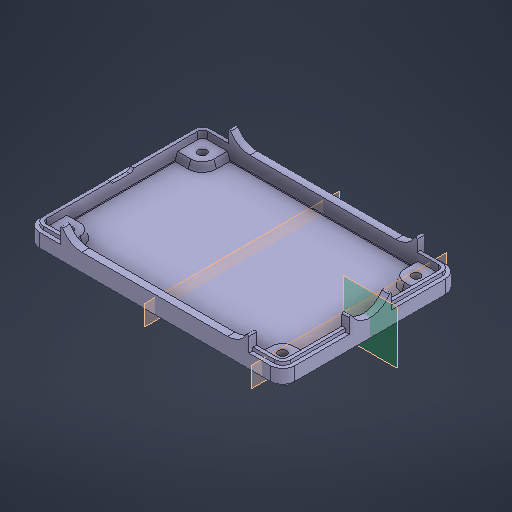
# Autodesk Inventor part: case1
Saved by Autodesk Inventor 2025.2 (Build 292293000, 293)
## iProperties
Created: 2025-10-04
Part Number: case1
Material: Generic
Document SubType Name: Modeling
Designer: micyg
Density: 1 g/cm^3
Appearance: Default
Author: micyg
## iProperties of the stored document case1_3DPrint.ipt
Created: 2025-10-05
Part Number: case1_3DPrint
Material: Generic
Document SubType Name: Modeling
Designer: micyg
Density: 1 g/cm^3
Appearance: Default
Author: micyg
Autodesk Inventor part; units mm, degrees
ref_plane "YZ Plane" through (0, 0, 0) normal (1, 0, 0) x (0, 1, 0)
ref_plane "XZ Plane" through (0, 0, 0) normal (0, 1, 0) x (-1, 0, 0)
ref_plane "XY Plane" through (0, 0, 0) normal (0, 0, 1) x (1, 0, 0)
sketch "Sketch1" plane through (0, 0, 0) normal (0, 1, 0) x (-1, 0, 0)
  line L0 (0, 0) -> (105.2, 0)
  line L1 (105.2, 0) -> (105.2, -72.2)
  line L2 (105.2, -72.2) -> (0, -72.2)
  line L3 (0, -72.2) -> (0, 0)
  line L4 (0, -72.2) -> (105.2, 0) construction
  line L5 (3.6, -3.6) -> (101.6, -3.6) construction
  line L6 (101.6, -3.6) -> (101.6, -68.6) construction
  line L7 (101.6, -68.6) -> (3.6, -68.6) construction
  line L8 (3.6, -68.6) -> (3.6, -3.6) construction
  line L9 (3.6, -3.6) -> (101.6, -68.6) construction
  line L10 (101.6, -3.6) -> (3.6, -68.6) construction
  point P0 (52.6, -36.1)
  dimension "d17" = 98
  dimension "d18" = 65
  dimension "d21" = 72.2
  dimension "d22" = 105.2
  constraints: 22 end point, 4 parallel, 3 midpoint, 2 horizontal, 2 perpendicular
  measures "d17" distance of L6.end L7.end
  measures "d18" distance of L5.end L6.end
  measures "d21" distance between parallel lines of L2 L0
  measures "d22" distance between parallel lines of L3 L1
extrude "Extrusion1" add sketch "Sketch1" along normal blind 7.6
ref_plane "Work Plane7" through (0, 7.6, -36.1) normal (0, 0, -1) x (-1, 0, 0)
fillet "Fillet3" radius 5 4 edges at (-105.2, 3.8, -72.2) (-105.2, 3.8, 0) (0, 3.8, -72.2) (0, 3.8, 0)
chamfer "Chamfer1" distance 2 angle 45 8 edges at (0, 0, -36.1) (-1.4645, 0, -70.7355) (-52.6, 0, -72.2) (-103.7355, 0, -70.7355) (-105.2, 0, -36.1) (-103.7355, 0, -1.4645) (-52.6, 0, 0) (-1.4645, 0, -1.4645)
shell "Shell2" thickness 3 removed faces 1 at (-36.7333, 7.6, -48.1333)
sketch "Sketch2" plane through (-100.2, 3, -69.2) normal (0, 1, 0) x (1, 0, 0)
  line L0 (91.5, -5.6) -> (3.5, -5.6) construction
  line L1 (3.5, -5.6) -> (3.5, -60.6) construction
  line L2 (3.5, -60.6) -> (91.5, -60.6) construction
  line L3 (91.5, -60.6) -> (91.5, -5.6) construction
  arc A0 (91.5, -55.85) -> (86.75, -60.6) centre (91.5, -60.6) ccw
  line L4 (95, 0) -> (0, 0) construction
  arc A1 (-2, -64.2) -> (0, -66.2) centre (0, -64.2) ccw projected
  line L5 (-2, -64.2) -> (-2, -2) projected
  arc A2 (0, 0) -> (-2, -2) centre (0, -2) ccw projected
  line L6 (0, 0) -> (95.2, 0) projected
  arc A3 (97.2, -2) -> (95.2, 0) centre (95.2, -2) ccw projected
  line L7 (97.2, -2) -> (97.2, -64.2) projected
  arc A4 (95.2, -66.2) -> (97.2, -64.2) centre (95.2, -64.2) ccw projected
  line L8 (95.2, -66.2) -> (0, -66.2) projected
  arc A5 (95.2, -69.2) -> (100.2, -64.2) centre (95.2, -64.2) ccw projected
  line L9 (100.2, -64.2) -> (100.2, -2) projected
  arc A6 (100.2, -2) -> (95.2, 3) centre (95.2, -2) ccw projected
  line L10 (95.2, 3) -> (0, 3) projected
  arc A7 (0, 3) -> (-5, -2) centre (0, -2) ccw projected
  line L11 (-5, -2) -> (-5, -64.2) projected
  arc A8 (-5, -64.2) -> (0, -69.2) centre (0, -64.2) ccw projected
  line L12 (0, -69.2) -> (95.2, -69.2) projected
  line L13 (91.5, -55.85) -> (97.2, -55.85)
  line L14 (86.75, -60.6) -> (86.75, -66.2)
  circle A9 centre (91.5, -60.6) radius 1.75
  line L15 (-5, -2) -> (-5, -64.2) projected
  line L16 (-5, -33.1) -> (100.2, -33.1) construction
  line L17 (47.6, -69.2) -> (47.6, 3) construction
  line L18 (3.5, -60.6) -> (91.5, -5.6) construction
  line L19 (47.5, -5.6) -> (47.5, -60.6) construction
  line L20 (-1.5, -0.6) -> (96.5, -0.6) construction
  line L21 (96.5, -0.6) -> (96.5, -65.6) construction
  line L22 (96.5, -65.6) -> (-1.5, -65.6) construction
  line L23 (-1.5, -65.6) -> (-1.5, -0.6) construction
  line L24 (-1.5, -0.6) -> (96.5, -65.6) construction
  arc A10 (86.75, -5.6) -> (91.5, -10.35) centre (91.5, -5.6) ccw
  line L25 (91.5, -10.35) -> (97.2, -10.35)
  line L26 (86.75, -5.6) -> (86.75, 0)
  circle A11 centre (91.5, -5.6) radius 1.75
  arc A12 (8.25, -60.6) -> (3.5, -55.85) centre (3.5, -60.6) ccw
  line L27 (8.25, -60.6) -> (8.25, -66.2)
  circle A13 centre (3.5, -60.6) radius 1.75
  arc A14 (3.5, -10.35) -> (8.25, -5.6) centre (3.5, -5.6) ccw
  line L28 (8.25, -5.6) -> (8.25, 0)
  circle A15 centre (3.5, -5.6) radius 1.75
  line L29 (3.5, -10.35) -> (-2, -10.35)
  line L30 (3.5, -55.85) -> (-2, -55.85)
  point P0 (100.2, -69.2)
  point P1 (47.5, -33.1)
  point P2 (47.5, -33.1)
  point P3 (97.2, -10.35)
  point P4 (8.25, 0)
  dimension "d13" = 88
  dimension "d14" = 55
  dimension "d25" = 3.5
  dimension "d26" = 3
  dimension "d73" = 65
  dimension "d74" = 98
  dimension "d75" = 0.5
  dimension "d76" = 0.7
  constraints: 42 end point, 16 symmetric about line, 9 midpoint, 9 point on circle, 8 centre point, 7 point on line, 4 parallel, 3 coincident, 3 perpendicular, 3 tangent, 2 horizontal, 6 other
  measures "d13" distance between parallel lines of L1 L3
  measures "d14" distance of L2.end L0.start
  measures "d25" diameter of A9
  measures "d26" radial gap between concentric circles of A0 A9
  measures "d73" distance of L20.end L21.end
  measures "d74" distance of L20.start L20.end
  measures "d75" distance between parallel lines of L5 L23
  measures "d76" distance between parallel lines of L21 L7
extrude "Extrusion2" add sketch "Sketch2" along normal blind 3 contours L13 L7 A4 L8 L14 A0 | L25 A10 L26 L6 A3 L7 | L8 A1 L5 L30 A12 L27 | L28 A14 L29 L5 A2 L6
ref_plane "Work Plane1" through (-52.6, 7.6, -3) normal (-1, 0, 0) x (0, -1, 0)
ref_plane "Work Plane2" through (-3, 7.6, -36.1) normal (0, 0, 1) x (1, 0, 0)
ref_plane "Work Plane5" through (-52.7, 3, -36.1) normal (1, 0, 0) x (0, 0, -1)
ref_plane "Work Plane6" through (-8.7, 3, -8.6) normal (1, 0, 0) x (0, 0, -1)
sketch "Sketch12" plane through (-8.7, 3, -8.6) normal (1, 0, 0) x (0, 0, -1)
  line L0 (0, 3) -> (-5.6, 3) projected
  line L1 (-3.6, 3) -> (-5.6, 3) projected
  line L2 (4.75, 3) -> (-3.6, 3) projected
  line L3 (4.75, 3) -> (0, 3) projected
  line L4 (-1.75, 3) -> (1.75, 3) projected
  line L5 (-1.75, 3) -> (1.75, 3) projected
  line L6 (1.75, 0) -> (-1.75, 0) projected
  line L7 (-1.75, 3) -> (-1.75, 0) projected
  line L8 (1.75, 3) -> (1.75, 0) projected
  line L9 (-8.6, 4.6) -> (-8.6, -1) projected
  line L10 (-8.6, -1) -> (-8.6, 4.6) projected
  line L11 (-1.75, 0) -> (-3, -1.25)
  line L12 (-3, -1.25) -> (-3, -3)
  line L13 (-1.75, 0) -> (0, 0)
  line L14 (-1.75, 0) -> (0, 0)
  line L15 (0, 0) -> (0, -3)
  line L16 (1.75, 0) -> (3, -1.25)
  line L17 (3, -1.25) -> (3, -3)
  line L18 (-6.6, -3) -> (-8.6, -1) projected
  line L19 (-8.6, -1) -> (-3.6, -1) projected
  line L20 (-3.6, -3) -> (-3.6, -1) projected
  line L21 (-3.6, -3) -> (-6.6, -3) projected
  line L22 (-3.6, -3) -> (-3.6, -1) projected
  line L23 (-3.6, -1) -> (58.6, -1) projected
  line L24 (58.6, -3) -> (58.6, -1) projected
  line L25 (58.6, -3) -> (-3.6, -3) projected
  line L26 (-8.6, -1) -> (-3.6, -1) projected
  line L27 (-8.6, -1) -> (-8.6, 4.6) projected
  line L28 (-8.6, 4.6) -> (-3.6, 4.6) projected
  line L29 (-3.6, 4.6) -> (-3.6, -1) projected
  point P0 (-8.6, -3)
  dimension "d77" = 45
  dimension "d78" = 6
  constraints: 14 end point, 3 symmetric about line, 2 point on line, 1 collinear, 1 midpoint, 1 perpendicular
  measures "d77" angle of L12 L11
  measures "d78" distance between parallel lines of L17 L12
revolve "Revolution2" cut sketch "Sketch12" angle 360 about axis through (-8.7, 3, -8.6) along (0, -1, 0) contours L16 L23 L15 L6 | L16 L17 L25 L15 L23
mirror "Mirror6" about plane through (-3, 7.6, -36.1) normal (0, 0, 1) of "Revolution2"
mirror "Mirror7" about plane through (-52.7, 3, -36.1) normal (1, 0, 0) of "Revolution2", "Mirror6"
draft "FaceDraft1" angle 20 pull direction (0, 1, 0) faces at (-11.075, 5, -12.7136) (-13.45, 5, -4.9475) (-4.9809, 5, -13.35) (-13.4367, 4, -63.245) (-4.9809, 5, -58.85) (-13.45, 5, -67.2525) (-92.7754, 5, -11.2758) (-100.2858, 5, -13.35) (-91.95, 5, -4.9475) (-94.9646, 5, -59.1783) (-91.95, 5, -67.2525) (-100.2858, 5, -58.85) fixed edges at (-12.0588, 6, -11.9588) (-13.45, 6, -5.8) (-5.85, 6, -13.35) (-12.0588, 6, -60.2412) (-5.85, 6, -58.85) (-13.45, 6, -66.4) (-93.3412, 6, -11.9588) (-99.45, 6, -13.35) (-91.95, 6, -5.8) (-93.3412, 6, -60.2412) (-91.95, 6, -66.4) (-99.45, 6, -58.85)
sketch "Sketch5" plane through (0, 7.6, 0) normal (0, 1, 0) x (1, 0, 0)
  arc A0 (-100.2, 69.2) -> (-102.2, 67.2) centre (-100.2, 67.2) ccw projected
  line L0 (-100.2, 69.2) -> (-5, 69.2) projected
  arc A1 (-3, 67.2) -> (-5, 69.2) centre (-5, 67.2) ccw projected
  line L1 (-3, 67.2) -> (-3, 5) projected
  arc A2 (-5, 3) -> (-3, 5) centre (-5, 5) ccw projected
  line L2 (-5, 3) -> (-100.2, 3) projected
  arc A3 (-102.2, 5) -> (-100.2, 3) centre (-100.2, 5) ccw projected
  line L3 (-102.2, 5) -> (-102.2, 67.2) projected
  arc A4 (-5, 0) -> (0, 5) centre (-5, 5) ccw projected
  line L4 (0, 5) -> (0, 67.2) projected
  arc A5 (0, 67.2) -> (-5, 72.2) centre (-5, 67.2) ccw projected
  line L5 (-5, 72.2) -> (-100.2, 72.2) projected
  arc A6 (-100.2, 72.2) -> (-105.2, 67.2) centre (-100.2, 67.2) ccw projected
  line L6 (-105.2, 67.2) -> (-105.2, 5) projected
  arc A7 (-105.2, 5) -> (-100.2, 0) centre (-100.2, 5) ccw projected
  line L7 (-100.2, 0) -> (-5, 0) projected
  arc A8 (-100.2, 70.6) -> (-103.6, 67.2) centre (-100.2, 67.2) ccw
  line L8 (-100.2, 70.6) -> (-5, 70.6)
  arc A9 (-1.6, 67.2) -> (-5, 70.6) centre (-5, 67.2) ccw
  line L9 (-1.6, 67.2) -> (-1.6, 5)
  arc A10 (-5, 1.6) -> (-1.6, 5) centre (-5, 5) ccw
  line L10 (-5, 1.6) -> (-100.2, 1.6)
  arc A11 (-103.6, 5) -> (-100.2, 1.6) centre (-100.2, 5) ccw
  line L11 (-103.6, 5) -> (-103.6, 67.2)
  point P0 (0, 0)
  dimension "d35" = 1.4
  constraints: 8 end point, 8 point on circle, 4 centre point, 7 other
  measures "d35" distance between parallel lines of L3 L11
extrude "Extrusion4" add sketch "Sketch5" along normal blind 1.4 contours L8 A9 L9 A10 L10 A11 L11 A8
sketch "Sketch15" plane through (-105.2, 7.6, -67.2) normal (-1, 0, 0) x (0, 0, 1)
  arc A0 (35.57, 2.615) -> (34.29, 3.895) centre (34.29, 2.615) ccw construction
  arc A1 (35.37, 2.615) -> (34.29, 3.695) centre (34.29, 2.615) ccw construction
  line L0 (31.1, 3.695) -> (34.29, 3.695) construction
  line L1 (31.1, 3.895) -> (34.29, 3.895)
  line L2 (35.57, 2.615) -> (35.57, 2.015) construction
  line L3 (35.37, 2.615) -> (35.37, 2.015) construction
  arc A2 (34.29, 0.935) -> (35.37, 2.015) centre (34.29, 2.015) ccw construction
  arc A3 (34.29, 0.735) -> (35.57, 2.015) centre (34.29, 2.015) ccw construction
  line L4 (34.29, 0.935) -> (31.1, 0.935) construction
  line L5 (34.29, 0.735) -> (31.1, 0.735) construction
  arc A4 (27.91, 3.695) -> (26.83, 2.615) centre (27.91, 2.615) ccw construction
  arc A5 (27.91, 3.895) -> (26.63, 2.615) centre (27.91, 2.615) ccw construction
  line L6 (31.1, 3.895) -> (27.91, 3.895)
  line L7 (31.1, 3.695) -> (27.91, 3.695) construction
  line L8 (26.63, 2.615) -> (26.63, 2.015) construction
  line L9 (26.83, 2.615) -> (26.83, 2.015) construction
  arc A6 (26.63, 2.015) -> (27.91, 0.735) centre (27.91, 2.015) ccw construction
  arc A7 (26.83, 2.015) -> (27.91, 0.935) centre (27.91, 2.015) ccw construction
  line L10 (27.91, 0.935) -> (31.1, 0.935) construction
  line L11 (27.91, 0.735) -> (31.1, 0.735) construction
  line L12 (31.1, 0.235) -> (34.29, 0.235)
  arc A8 (34.29, 0.235) -> (36.07, 2.015) centre (34.29, 2.015) ccw
  line L13 (36.07, 2.015) -> (36.07, 2.615)
  arc A9 (36.07, 2.615) -> (34.29, 4.395) centre (34.29, 2.615) ccw
  line L14 (34.29, 4.395) -> (31.1, 4.395)
  line L15 (31.1, 4.395) -> (27.91, 4.395)
  arc A10 (27.91, 4.395) -> (26.13, 2.615) centre (27.91, 2.615) ccw
  line L16 (26.13, 2.615) -> (26.13, 2.015)
  arc A11 (26.13, 2.015) -> (27.91, 0.235) centre (27.91, 2.015) ccw
  line L17 (27.91, 0.235) -> (31.1, 0.235)
  point P0 (67.2, -7.6)
  dimension "d84" = 0.5
  constraints: 36 end point, 24 point on circle, 12 centre point, 8 horizontal, 4 vertical, 45 other
  measures "d84" distance between parallel lines of L5 L12
extrude "Extrusion10" cut sketch "Sketch15" against normal up to surface (3 mm away)
sketch "Sketch17" plane through (-100.2, 7.6, 0) normal (0, 0, 1) x (1, 0, 0)
  circle A0 centre (17.5, 10.585) radius 7 construction
  circle A1 centre (37.5, 10.585) radius 7 construction
  circle A2 centre (57.5, 10.585) radius 7 construction
  circle A3 centre (77.5, 10.585) radius 7 construction
  circle A4 centre (17.5, 10.585) radius 9
  circle A5 centre (37.5, 10.585) radius 9 construction
  circle A6 centre (57.5, 10.585) radius 9 construction
  circle A7 centre (77.5, 10.585) radius 9
  line L0 (8.5, 10.585) -> (86.5, 10.585) construction
  line L1 (86.5, 10.585) -> (86.5, 0)
  line L2 (86.5, 0) -> (8.5, 0)
  line L3 (8.5, 0) -> (8.5, 10.585)
  line L4 (95.2, 0) -> (95.2, -5.6) construction
  line L5 (0, 0) -> (95.2, 0) projected
  line L6 (0, -5.6) -> (0, 0) construction
  line L7 (0, 0) -> (95.2, 0) projected
  line L8 (17.5, 19.585) -> (77.5, 19.585)
  line L9 (77.5, 19.585) -> (77.5, 1.585) construction
  line L10 (77.5, 1.585) -> (17.5, 1.585)
  line L11 (17.5, 1.585) -> (17.5, 19.585) construction
  line L12 (8.7, 8.6982) -> (86.3, 8.6982) construction
  line L13 (86.3, 8.6982) -> (86.3, 0)
  line L14 (86.3, 0) -> (8.7, 0)
  line L15 (8.7, 0) -> (8.7, 8.6982)
  line L16 (95.2, -5.6) -> (0, -5.6) projected
  point P0 (100.2, -7.6)
  point P1 (17.5, 1.585)
  point P2 (8.7, 0)
  dimension "d87" = 18
  dimension "d88" = 18
  dimension "d89" = 18
  dimension "d90" = 18
  dimension "d97" = 0.2
  constraints: 24 end point, 8 centre point, 6 parallel, 5 coincident, 5 point on circle, 3 horizontal, 3 perpendicular, 3 point on line, 2 midpoint, 8 other
  measures "d87" diameter of A4
  measures "d88" diameter of A5
  measures "d89" diameter of A6
  measures "d90" diameter of A7
  measures "d97" distance between parallel lines of L3 L15
extrude "Extrusion11" add sketch "Sketch17" against normal up to surface (3 mm away) contours L10 A7 L13 L2 L15 A4
fillet "Fillet8" radius 0.5 2 edges at (-13.9, 16.2982, -1.5) (-91.5, 16.2982, -1.5)
mirror "Mirror8" about plane through (0, 7.6, -36.1) normal (0, 0, -1) of "Extrusion11", "Fillet8"
sketch "Sketch18" plane through (0, 7.6, -5) normal (1, 0, 0) x (0, 0, -1)
  line L0 (41.1, 0.585) -> (21.1, 0.585) construction
  line L1 (41.1, 0.585) -> (41.1, 20.085) construction
  line L2 (21.1, 20.085) -> (41.1, 20.085) construction
  line L3 (21.1, 20.085) -> (21.1, 0.585) construction
  circle A0 centre (31.1, 10.585) radius 7 construction
  circle A1 centre (31.1, 10.585) radius 9
  line L4 (0, 0) -> (62.2, 0) projected
  line L5 (22.1, 10.585) -> (40.1, 10.585)
  line L6 (40.1, 10.585) -> (40.1, 0)
  line L7 (40.1, 0) -> (22.1, 0)
  line L8 (22.1, 0) -> (22.1, 10.585)
  line L9 (22.4, 0) -> (39.8, 0)
  line L10 (39.8, 0) -> (39.8, 8.2807)
  line L11 (39.8, 8.2807) -> (22.4, 8.2807)
  line L12 (22.4, 8.2807) -> (22.4, 0)
  point P0 (-5, -7.6)
  point P1 (22.1, 0)
  point P2 (22.4, 0)
  point P3 (39.8, 0)
  dimension "d93" = 18
  dimension "d96" = 0.3
  constraints: 16 end point, 4 parallel, 4 point on circle, 2 horizontal, 2 perpendicular, 2 point on line, 1 centre point, 1 coincident, 1 midpoint
  measures "d93" diameter of A1
  measures "d96" distance between parallel lines of L12 L8
extrude "Extrusion12" add sketch "Sketch18" against normal up to surface (3 mm away) contours L10 L4 L12 A1
fillet "Fillet7" radius 0.5 2 edges at (-1.5, 15.8807, -27.4) (-1.5, 15.8807, -44.8)
body "Solid1"
